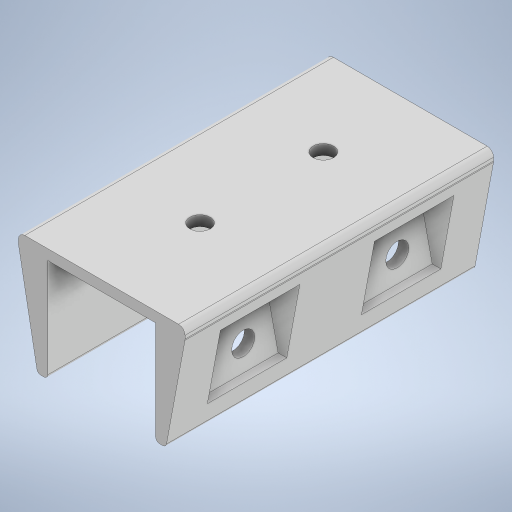
# Autodesk Inventor part: Motor Controller Mount
Saved by Autodesk Inventor 2024.1 (Build 281209000, 209)
## iProperties
Created: 2024-01-25
Part Number: Motor Controller Mount
Material: Generic
Document SubType Name: Modeling
Designer: dbt5238
Density: 1 g/cm^3
Appearance: Default
Author: dbt5238
Autodesk Inventor part; units mm, degrees
ref_plane "YZ Plane" through (0, 0, 0) normal (1, 0, 0) x (0, 1, 0)
ref_plane "XZ Plane" through (0, 0, 0) normal (0, 1, 0) x (-1, 0, 0)
ref_plane "XY Plane" through (0, 0, 0) normal (0, 0, 1) x (1, 0, 0)
sketch "Sketch1" plane through (0, 0, 0) normal (0, 1, 0) x (-1, 0, 0)
  circle A0 centre (-16.22, -19.1467) radius 1.7294
  circle A1 centre (-16.22, -43.1467) radius 1.7294
  line L0 (0, 0) -> (-32.44, 0)
  line L1 (-32.44, 0) -> (-32.44, -60.0777)
  line L2 (-32.44, -60.0777) -> (0, -60.0777)
  line L3 (0, -60.0777) -> (0, 0)
  point P0 (-16.22, 0)
  dimension "d27" = 24
  dimension "d28" = 60.0777
  dimension "d29" = 32.44
  dimension "d30" = 19.1467
  dimension "d31" = 16.22
  dimension "d32" = 3.4587
  constraints: 8 end point, 2 centre point, 2 parallel, 1 coincident, 1 equal radius, 1 horizontal, 1 midpoint, 1 perpendicular, 1 vertical alignment
  measures "d27" distance of A1.centre A0.centre
  measures "d28" distance between parallel lines of L2 L0
  measures "d29" distance between parallel lines of L1 L3
  measures "d30" distance of point (-16.22, 0) A0.centre
  measures "d31" distance from line of L3 A0.centre
  measures "d32" diameter of A0
extrude "Extrusion2" add sketch "Sketch1" along normal blind 2
sketch "Sketch2" plane through (0, 2, 0) normal (0, 1, 0) x (1, 0, 0)
  circle A0 centre (16.22, 43.1467) radius 1.7294 projected
  circle A1 centre (16.22, 19.1467) radius 1.7294 projected
  circle A2 centre (16.22, 43.1467) radius 1.7294 projected
  line L0 (32.44, 0) -> (0, 0) projected
  line L1 (0, 0) -> (0, 60.0777) projected
  line L2 (0, 60.0777) -> (32.44, 60.0777) projected
  line L3 (32.44, 60.0777) -> (32.44, 0) projected
  constraints: 2 coincident
hole "Hole1" at (16.22, 2, -43.1467) at (16.22, 2, -19.1467) direction (0, -1, 0) diameter 4 end through all
sketch "Sketch3" plane through (0, 0, 0) normal (0, 0, 1) x (1, 0, 0)
  line L0 (32.44, 0) -> (0, 0) projected
  line L1 (28.72, 0) -> (26.72, 0)
  line L2 (26.72, 0) -> (26.72, -20)
  line L3 (26.72, -20) -> (28.72, -20)
  line L4 (28.72, -20) -> (28.72, 0)
  line L5 (16.22, 0) -> (16.22, -9.2912) construction
  line L6 (3.72, 0) -> (5.72, 0)
  line L7 (5.72, 0) -> (5.72, -20)
  line L8 (5.72, -20) -> (3.72, -20)
  line L9 (3.72, -20) -> (3.72, 0)
  line L10 (28.72, -20) -> (32.44, 0)
  line L11 (28.72, 0) -> (32.44, 0)
  line L12 (3.72, -20) -> (3.72, 0)
  line L13 (3.72, -20) -> (0, 0)
  line L14 (3.72, 0) -> (0, 0)
  dimension "d42" = 10.5
  dimension "d43" = 2
  dimension "d44" = 20
  constraints: 28 end point, 4 symmetric about line, 2 parallel, 1 collinear, 1 horizontal, 1 midpoint, 1 perpendicular, 1 point on line, 1 vertical
  measures "d42" distance from line of L2 L5.start
  measures "d43" distance between parallel lines of L4 L2
  measures "d44" distance between parallel lines of L0 L3
extrude "Extrusion3" add sketch "Sketch3" against normal up to surface (60.0777 mm away)
fillet "Fillet1" radius 0.75 4 edges at (3.72, -20, -30.0389) (5.72, -20, -30.0389) (28.72, -20, -30.0389) (26.72, -20, -30.0389)
fillet "Fillet2" radius 1.25 4 edges at (32.44, 0, -30.0389) (0, 0, -30.0389) (0, 2, -30.0389) (32.44, 2, -30.0389)
ref_plane "Work Plane3" through (5.72, 0, -15.0389) normal (0, 0, 1) x (1, 0, 0)
ref_plane "Work Plane2" through (5.72, 0, -30.0389) normal (0, 0, 1) x (1, 0, 0)
sketch "Sketch4" plane through (5.72, 0, -15.0389) normal (0, 0, 1) x (1, 0, 0)
  arc A0 (-0.75, -20) -> (0, -19.25) centre (-0.75, -19.25) ccw projected
  line L0 (-0.75, -20) -> (-1.3766, -20) projected
  arc A1 (-2.114, -19.3871) -> (-1.3766, -20) centre (-1.3766, -19.25) ccw projected
  line L1 (-2.114, -19.3871) -> (-5.6989, -0.1133) projected
  arc A2 (-5.72, 0.1153) -> (-5.6989, -0.1133) centre (-4.47, 0.1153) ccw projected
  line L2 (-5.72, 0.1153) -> (-5.72, 0.75) projected
  arc A3 (-4.47, 2) -> (-5.72, 0.75) centre (-4.47, 0.75) ccw projected
  line L3 (-4.47, 2) -> (25.47, 2) projected
  arc A4 (26.72, 0.75) -> (25.47, 2) centre (25.47, 0.75) ccw projected
  line L4 (26.72, 0.75) -> (26.72, 0.1153) projected
  arc A5 (26.6989, -0.1133) -> (26.72, 0.1153) centre (25.47, 0.1153) ccw projected
  line L5 (26.6989, -0.1133) -> (23.114, -19.3871) projected
  arc A6 (22.3766, -20) -> (23.114, -19.3871) centre (22.3766, -19.25) ccw projected
  line L6 (22.3766, -20) -> (21.75, -20) projected
  arc A7 (21, -19.25) -> (21.75, -20) centre (21.75, -19.25) ccw projected
  line L7 (21, -19.25) -> (21, 0) projected
  line L8 (21, 0) -> (0, 0) projected
  line L9 (0, 0) -> (0, -19.25) projected
  line L10 (23, 0) -> (23, -19.667)
  line L11 (23, -5) -> (25.79, -5)
  line L12 (25.79, -5) -> (23.93, -15)
  line L13 (23, -15) -> (23.93, -15)
  point P0 (-5.72, 0)
  point P1 (24.86, -10)
  dimension "d51" = 2
  dimension "d52" = 10
  dimension "d53" = 5
  constraints: 8 end point, 4 point on line, 2 parallel, 1 midpoint, 1 point on circle, 1 vertical
  measures "d51" distance between parallel lines of L7 L10
  measures "d52" distance from line of L8 point (24.86, -10)
  measures "d53" distance from line of point (24.86, -10) L11
extrude "Extrusion4" cut sketch "Sketch4" along normal mid plane 10 contours L10 L11 L5 L13
sketch "Sketch5" plane through (28.72, -15, -20.0389) normal (1, 0, 0) x (0, 0, -1)
  line L0 (-10, 10) -> (0, 10) projected
  line L1 (-10, 0) -> (-10, 10) projected
  point P0 (-20.0389, 15)
  point P1 (-5, 5)
  dimension "d63" = 5
  dimension "d64" = 5
  measures "d63" distance from line of L0 point (-5, 5)
  measures "d64" distance from line of L1 point (-5, 5)
hole "Hole2" at (28.72, -10, -15.0389) direction (-1, 0, 0) diameter 4.5 depth 2 tip angle 118 clearance for "Socket Head Cap Screw" size "M4" standard "Ansi Metric M Profile"
ref_plane "Work Plane4" through (16.22, 0, 0) normal (1, 0, 0) x (0, 0, -1)
mirror "Mirror2" about plane through (16.22, 0, 0) normal (1, 0, 0) of "Extrusion4", "Hole2"
mirror "Mirror3" about plane through (5.72, 0, -30.0389) normal (0, 0, 1) of "Extrusion4", "Hole2", "Mirror2"
chamfer "Chamfer1" distance 2.73 angle 45 8 edges at (30.58, -10, -10.0389) (30.58, -10, -20.0389) (30.58, -10, -50.0389) (30.58, -10, -40.0389) (1.86, -10, -10.0389) (1.86, -10, -20.0389) (1.86, -10, -40.0389) (1.86, -10, -50.0389)
chamfer "Chamfer2" distance 2.79 angle 45 4 edges at (31.51, -5, -15.0389) (31.51, -5, -45.0389) (0.93, -5, -15.0389) (0.93, -5, -45.0389)
chamfer "Chamfer3" distance 0.93 angle 45 4 edges at (29.65, -15, -15.0389) (2.79, -15, -15.0389) (2.79, -15, -45.0389) (29.65, -15, -45.0389)
body "Solid2"
